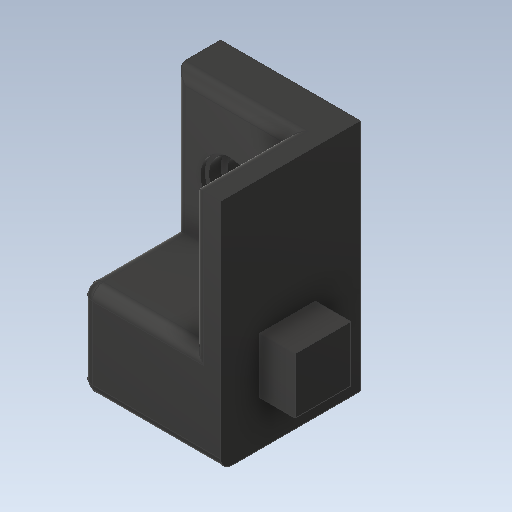
# Autodesk Inventor part: frame-holder-v3
Saved by Autodesk Inventor 2020 (Build 240168000, 168)
## iProperties
Created: 2018-02-27
Part Number: frame-holder-v3
Material: 一般
Document SubType Name: Modeling
Designer: qiuyu
Density: 1 g/cm^3
Appearance: Smooth - Black
Mass: 17.9644 g
Surface Area: 61.8477 cm^2
Volume: 17.9644 cm^3
Author: qiuyu
Autodesk Inventor part; units mm, degrees
ref_plane "YZ Plane" through (0, 0, 0) normal (1, 0, 0) x (0, 1, 0)
ref_plane "XZ Plane" through (0, 0, 0) normal (0, 1, 0) x (-1, 0, 0)
ref_plane "XY Plane" through (0, 0, 0) normal (0, 0, 1) x (1, 0, 0)
sketch "Sketch1" plane through (0, 0, 0) normal (1, 0, 0) x (0, 1, 0)
  line L0 (-8.5, 12.5) -> (8.5, 12.5)
  line L1 (8.5, 12.5) -> (8.5, -12.5)
  line L2 (8.5, -12.5) -> (-8.5, -12.5)
  line L3 (-8.5, -12.5) -> (-8.5, 12.5)
  line L4 (-8.5, 12.5) -> (8.5, -12.5) construction
  line L5 (8.5, 12.5) -> (-8.5, -12.5) construction
  line L6 (8.5, -12.5) -> (33.5, -12.5)
  line L7 (8.5, -12.5) -> (33.5, -12.5) construction
  line L8 (33.5, -12.5) -> (33.5, -4.25)
  line L9 (33.5, -4.25) -> (8.5, -4.25)
  line L10 (33.5, -4.25) -> (58.5, -4.25) construction
  point P0 (0, 0)
  dimension "d0" = 17
  dimension "d1" = 25
  dimension "d2" = 25
  dimension "d3" = 0
  dimension "d4" = 8.25
  dimension "d5" = 90
  dimension "d6" = 180
  constraints: 22 end point, 4 horizontal, 2 collinear, 2 midpoint, 2 parallel, 2 perpendicular, 1 point on line
  measures "d0" distance of L1.end L2.end
  measures "d1" distance of L0.end L1.end
  measures "d2" distance of L1.end L6.end
  measures "d3" distance between parallel lines of L6 L7
  measures "d4" distance of L6.end L8.end
  measures "d5" angle of L8 L6
  measures "d6" angle of L9 L10
extrude "Extrusion1" add sketch "Sketch1" along normal blind 20
sketch "Sketch2" plane through (0, 8.5, -4.25) normal (0, 0, 1) x (1, 0, 0)
  circle A0 centre (10, 10.5) radius 3.81
  line L0 (0, 25) -> (20, 25) projected
  line L1 (0, -8.5) -> (20, -8.5) construction
  line L2 (20, -17) -> (20, 25) projected
  dimension "d9" = 7.62
  dimension "d32" = 19
  constraints: 2 end point, 1 centre point, 1 horizontal, 1 point on line
  measures "d9" diameter of A0
  measures "d32" distance from line of L1 A0.centre
extrude "Extrusion2" cut sketch "Sketch2" against normal through all
sketch "Sketch3" plane through (0, 8.5, -4.25) normal (0, 0, 1) x (1, 0, 0)
  circle A0 centre (10, 10.5) radius 3.81 projected
  circle A1 centre (10, 10.5) radius 4.815
  point P0 (0, -8.5)
  dimension "d13" = 9.63
  constraints: 1 centre point, 1 coincident
  measures "d13" diameter of A1
extrude "Extrusion3" cut sketch "Sketch3" against normal blind 3.2
sketch "Sketch4" plane through (0, 8.5, -4.25) normal (0, 0, 1) x (1, 0, 0)
  circle A0 centre (10, 10.5) radius 3.81 projected
  circle A1 centre (10, 10.5) radius 5.39
  point P0 (0, -8.5)
  dimension "d16" = 10.78
  constraints: 1 centre point, 1 coincident
  measures "d16" diameter of A1
extrude "Extrusion4" cut sketch "Sketch4" against normal blind 0.92
sketch "Sketch6" plane through (0, -8.5, -12.5) normal (0, -1, 0) x (1, 0, 0)
  circle A0 centre (10, 12) radius 6.2485
  line L0 (0, 0) -> (20, 0) projected
  line L1 (0, 25) -> (0, 0) projected
  point P0 (0, 12.5)
  dimension "d22" = 12.497
  dimension "d25" = 12
  dimension "d26" = 10
  constraints: 1 centre point
  measures "d22" diameter of A0
  measures "d25" distance from line of A0.centre L0
  measures "d26" distance from line of A0.centre L1
extrude "Extrusion6" [suppressed]
sketch "Sketch9" plane through (0, -8.5, -12.5) normal (0, 0, -1) x (-1, 0, 0)
  line L0 (-5, 20) -> (-15, 20)
  line L1 (-15, 20) -> (-15, 10)
  line L2 (-15, 10) -> (-5, 10)
  line L3 (-5, 10) -> (-5, 20)
  line L4 (0, 0) -> (0, 42) projected
  line L5 (0, 0) -> (-20, 0) projected
  point P0 (0, 8.5)
  dimension "d38" = 10
  dimension "d39" = 10
  dimension "d40" = 5
  dimension "d41" = 10
  constraints: 8 end point, 2 parallel, 1 horizontal, 1 perpendicular
  measures "d38" distance of L2.end L1.end
  measures "d39" distance of L1.end L0.end
  measures "d40" distance between parallel lines of L4 L3
  measures "d41" distance between parallel lines of L5 L2
extrude "Extrusion8" add sketch "Sketch9" along normal blind 6.35
sketch "Sketch12" plane through (20, 0, 0) normal (1, 0, 0) x (0, 0, -1)
  line L0 (12.5, -8.5) -> (12.5, 33.5) projected
  line L1 (12.5, 33.5) -> (4.25, 33.5) projected
  line L2 (4.25, 33.5) -> (4.25, 8.5) projected
  line L3 (4.25, 8.5) -> (-12.5, 8.5) projected
  line L4 (-12.5, 8.5) -> (-12.5, -8.5) projected
  line L5 (-12.5, -8.5) -> (12.5, -8.5) projected
  line L6 (-12.5, -8.5) -> (12.5, -8.5) projected
  line L7 (12.5, -8.5) -> (-12.5, -8.5)
  line L8 (-12.5, -8.5) -> (-12.5, 33.5)
  line L9 (-12.5, 33.5) -> (12.5, 33.5)
  line L10 (12.5, 33.5) -> (12.5, -8.5)
  line L11 (12.5, 33.5) -> (4.25, 33.5) projected
  line L12 (-12.5, 8.5) -> (-12.5, -8.5) projected
  point P0 (0, 0)
  constraints: 8 end point, 2 collinear, 2 parallel, 1 horizontal, 1 perpendicular
extrude "Extrusion10" add sketch "Sketch12" along normal blind 5
sketch "Sketch14" plane through (0, 0, 0) normal (-1, 0, 0) x (0, 0, 1)
  circle A0 centre (3.3578, 0) radius 4.1
  line L0 (-12.5, -8.5) -> (-12.5, 33.5) projected
  line L1 (12.5, -8.5) -> (-12.5, -8.5) projected
  line L2 (12.5, 8.5) -> (12.5, -8.5) projected
  line L3 (-4.25, 8.5) -> (12.5, 8.5) projected
  line L4 (-4.25, 33.5) -> (-4.25, 8.5) projected
  line L5 (-12.5, 33.5) -> (-4.25, 33.5) projected
  point P0 (0, 0)
  dimension "d52" = 8.5
  dimension "d53" = 8.2
  constraints: 1 centre point
  measures "d52" distance from line of L3 A0.centre
  measures "d53" diameter of A0
extrude "Extrusion11" cut sketch "Sketch14" against normal blind 10.2 contours A0
sketch "Sketch15" plane through (25, 0, 0) normal (1, 0, 0) x (0, 0, -1)
  line L0 (12.5, -8.5) -> (12.5, 33.5) projected
  line L1 (12.5, 33.5) -> (-12.5, 33.5) projected
  line L2 (-12.5, 33.5) -> (-12.5, -8.5) projected
  line L3 (-12.5, -8.5) -> (12.5, -8.5) projected
  circle A0 centre (-3.3578, 0) radius 4.1 projected
  circle A1 centre (-3.3578, 0) radius 4.1 projected
  line L4 (-5.5, -0.5) -> (4.5, -0.5)
  line L5 (4.5, -0.5) -> (4.5, 9.5)
  line L6 (4.5, 9.5) -> (-5.5, 9.5)
  line L7 (-5.5, 9.5) -> (-5.5, -0.5)
  line L8 (-5.5, -0.5) -> (4.5, 9.5) construction
  line L9 (4.5, -0.5) -> (-5.5, 9.5) construction
  point P0 (0, 0)
  point P1 (-0.5, 4.5)
  dimension "d56" = 10
  dimension "d57" = 10
  dimension "d58" = 8
  dimension "d59" = 8
  constraints: 12 end point, 2 midpoint, 2 parallel, 1 horizontal, 1 perpendicular
  measures "d56" distance of L6.end L5.end
  measures "d57" distance of L5.end L4.end
  measures "d58" distance between parallel lines of L3 L4
  measures "d59" distance between parallel lines of L0 L5
extrude "Extrusion12" add sketch "Sketch15" along normal blind 6.35 contours A0 L4 L7 | A0 L7 L6 L5 L4 picked at (-1.3763, 0.1524)
fillet "Fillet3" radius 2 9 edges at (0, 21, -4.25) (0, 8.5, 4.125) (10, 8.5, 12.5) (0, 0, 12.5) (20, 21, 12.5) (20, 33.5, 4.125) (10, 33.5, -4.25) (12.5, -8.5, 12.5) (0, -8.5, 0)
sketch "Sketch10" plane through (0, 0, 0) normal (-1, 0, 0) x (0, 0, 1)
  line L0 (-12.5, -8.5) -> (-12.5, 33.5) projected
  line L1 (12.5, -8.5) -> (-12.5, -8.5) projected
  line L2 (12.5, 8.5) -> (12.5, -8.5) projected
  line L3 (-4.25, 8.5) -> (12.5, 8.5) projected
  line L4 (-4.25, 33.5) -> (-4.25, 8.5) projected
  line L5 (-12.5, 33.5) -> (-4.25, 33.5) projected
  line L6 (2.5, 6.5) -> (-7.5, 6.5)
  line L7 (-7.5, 6.5) -> (-7.5, -3.5)
  line L8 (-7.5, -3.5) -> (2.5, -3.5)
  line L9 (2.5, -3.5) -> (2.5, 6.5)
  point P0 (0, 0)
  dimension "d44" = 10
  dimension "d45" = 10
  dimension "d46" = 5
  dimension "d47" = 5
  constraints: 8 end point, 2 parallel, 1 horizontal, 1 perpendicular
  measures "d44" distance of L8.end L7.end
  measures "d45" distance of L7.end L6.end
  measures "d46" distance between parallel lines of L7 L0
  measures "d47" distance between parallel lines of L1 L8
sketch "Sketch8" plane through (20, 0, 0) normal (1, 0, 0) x (0, 0, -1)
  circle A0 centre (-2, 0) radius 4.05
  line L0 (4.25, 13.61) -> (4.25, 24.39) projected
  line L1 (4.25, 10.5) -> (4.25, 31.5) projected
  line L2 (4.25, 31.5) -> (4.25, 10.5) projected
  line L3 (7.45, 22.81) -> (7.45, 15.19) projected
  line L4 (12.5, 22.81) -> (12.5, 15.19) projected
  line L5 (7.45, 22.81) -> (7.45, 15.19) projected
  point P0 (0, 0)
  dimension "d34" = 8.1
  dimension "d35" = 6.25
  constraints: 1 centre point, 1 horizontal alignment
  measures "d34" diameter of A0
  measures "d35" distance from line of A0.centre L0
sketch "Sketch5" plane through (20, 0, 0) normal (1, 0, 0) x (0, 0, -1)
  circle A0 centre (0, 0) radius 4.05
  line L0 (27.5, -8.5) -> (27.5, 33.5) projected
  line L1 (27.5, 33.5) -> (19.5, 33.5) projected
  line L2 (19.5, 33.5) -> (19.5, 8.5) projected
  line L3 (19.5, 8.5) -> (-27.5, 8.5) projected
  line L4 (-27.5, 8.5) -> (-27.5, -8.5) projected
  line L5 (-27.5, -8.5) -> (27.5, -8.5) projected
  dimension "d19" = 8.1
  dimension "d33" = 27.5
  constraints: 1 centre point, 1 coincident
  measures "d19" diameter of A0
  measures "d33" distance from line of point (0, 0) L0
body "Solid1"
